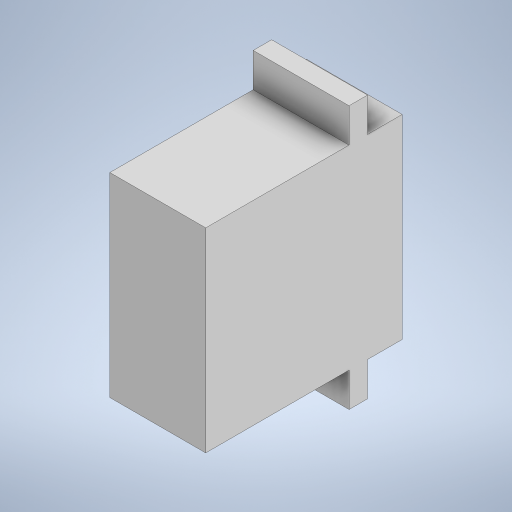
# Autodesk Inventor part: ServoSimplified
Saved by Autodesk Inventor 2024 (Build 280153000, 153)
## iProperties
Created: 2025-02-07
Part Number: ServoSimplified
Material: Generic
Document SubType Name: Modeling
Designer: Tommy Rohmann
Density: 1 g/cm^3
Appearance: Default
Author: Tommy Rohmann
Autodesk Inventor part; units mm, degrees
ref_plane "YZ Plane" through (0, 0, 0) normal (1, 0, 0) x (0, 1, 0)
ref_plane "XZ Plane" through (0, 0, 0) normal (0, 1, 0) x (-1, 0, 0)
ref_plane "XY Plane" through (0, 0, 0) normal (0, 0, 1) x (1, 0, 0)
sketch "Sketch1" plane through (0, 0, 0) normal (0, 0, 1) x (1, 0, 0)
  line L0 (0, 0) -> (19.7866, 0)
  line L1 (19.7866, 0) -> (19.7866, 40.2336)
  line L2 (19.7866, 40.2336) -> (0, 40.2336)
  line L3 (0, 40.2336) -> (0, 0)
  line L4 (0, 0) -> (19.7866, 0)
  line L5 (19.7866, 0) -> (19.7866, -7.0358)
  line L6 (19.7866, -7.0358) -> (0, -7.0358)
  line L7 (0, -7.0358) -> (0, 0)
  line L8 (19.7866, 20.1168) -> (0, 20.1168) construction
  line L9 (19.7866, 40.2336) -> (19.7866, 47.2694)
  line L10 (19.7866, 47.2694) -> (0, 47.2694)
  line L11 (0, 47.2694) -> (0, 40.2336)
  dimension "d0" = 19.7866
  dimension "d1" = 40.2336
  dimension "d2" = 7.0358
  constraints: 24 end point, 4 parallel, 3 symmetric about line, 2 horizontal, 2 midpoint, 2 perpendicular, 1 point on line
  measures "d0" distance of L2.end L1.end
  measures "d1" distance of L1.end L0.end
  measures "d2" distance of L4.end L5.end
extrude "Extrusion1" add sketch "Sketch1" along normal blind 29.591 contours L3 L2 L1 L0
extrude "Extrusion2" add sketch "Sketch1" against normal blind 3.81 contours L0 L5 L6 L7 | L11 L10 L9 L2
extrude "Extrusion3" add sketch "Sketch1" against normal blind 10.9601 contours L3 L2 L1 L0
body "Solid1"
